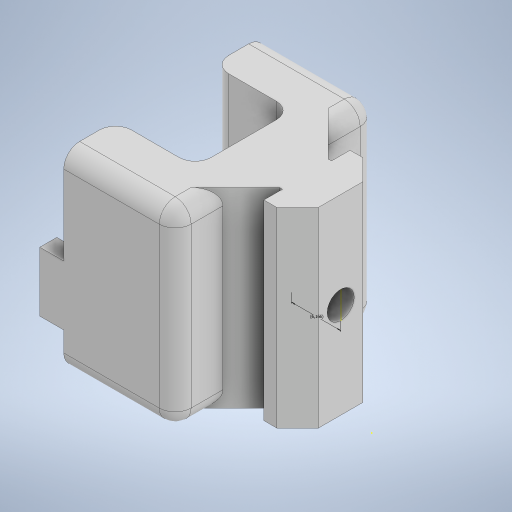
# Autodesk Inventor part: Montaż_kamery
Saved by Autodesk Inventor 2023 (Build 270158000, 158)
## iProperties
Created: 2023-04-17
Part Number: Montaż_kamery
Material: Ogólny
Document SubType Name: Modeling
Designer: janek
Density: 1 g/cm^3
Appearance: Domyślna
Author: janek
## iProperties of the stored document Montaż_kamery_Drukowanie 3D.ipt
Created: 2023-04-17
Part Number: Montaż_kamery_Drukowanie 3D
Material: Ogólny
Document SubType Name: Modeling
Designer: janek
Density: 1 g/cm^3
Appearance: Domyślna
Author: janek
Autodesk Inventor part; units mm, degrees
ref_plane "YZ Plane" through (0, 0, 0) normal (1, 0, 0) x (0, 1, 0)
ref_plane "XZ Plane" through (0, 0, 0) normal (0, 1, 0) x (-1, 0, 0)
ref_plane "XY Plane" through (0, 0, 0) normal (0, 0, 1) x (1, 0, 0)
sketch "Szkic3" plane through (0, 0, 0) normal (0, 1, 0) x (-1, 0, 0)
  line L0 (3.9, 2.7912) -> (3.9, -2.7912)
  line L1 (6.5152, 5.4063) -> (3.9, 2.7912)
  line L2 (8.1306, 5.4063) -> (6.5152, 5.4063)
  line L3 (8.1306, 5.4063) -> (8.1306, 3.0781)
  line L4 (8.1306, -3.0781) -> (8.1306, -5.4064)
  line L5 (8.1306, -5.4064) -> (6.5152, -5.4064)
  line L6 (6.5152, -5.4064) -> (3.9, -2.7912)
  line L7 (8.1306, 3.0781) -> (8.5306, 3.0781)
  line L8 (8.1306, -3.0781) -> (8.5306, -3.0781)
  line L9 (8.5306, -3.0781) -> (12.0661, -6.6136)
  line L10 (8.5306, 3.0781) -> (12.0661, 6.6136)
  line L11 (12.0661, -6.6136) -> (12.0661, -12.6136)
  line L12 (12.0661, 6.6136) -> (12.0661, 12.6136)
  line L13 (12.0661, 12.6136) -> (16.0661, 12.6136)
  line L14 (12.0661, -12.6136) -> (16.0661, -12.6136)
  line L15 (16.0661, -12.6136) -> (16.0661, 12.6136)
  point P0 (8.1306, 4.2422)
  dimension "d85" = 5.5823
  dimension "d88" = 135
  dimension "d89" = 135
  dimension "d90" = 1.6154
  dimension "d91" = 2.6152
  dimension "d92" = 2.3282
  dimension "d99" = 0.4
  dimension "d100" = 5
  dimension "d101" = 135
  dimension "d102" = 5
  dimension "d103" = 135
  dimension "d114" = 180
  dimension "d115" = 6
  dimension "d116" = 6
  dimension "d117" = 4
  dimension "d118" = 4
  constraints: 32 end point, 5 vertical, 4 equal length, 4 horizontal, 1 midpoint, 1 perpendicular, 1 other
  measures "d85" distance of L0.start L0.end
  measures "d88" angle of L6 L0
  measures "d89" angle of L1 L0
  measures "d90" distance of L4.end L5.end
  measures "d91" horizontal distance of L5.end L0.end
  measures "d92" distance of L4.start L4.end
  measures "d99" distance of L3.end L7.end
  measures "d100" distance of L8.end L9.end
  measures "d101" angle of L9 L8
  measures "d102" distance of L7.end L10.end
  measures "d103" angle of L7 L10
  measures "d114" angle of L2 L5
  measures "d115" distance of L9.end L11.end
  measures "d116" distance of L10.end L12.end
  measures "d117" distance of L12.end L13.end
  measures "d118" distance of L11.end L14.end
extrude "Wyciągnięcie proste1" add sketch "Szkic3" along normal blind 24
sketch "Szkic13" plane through (-16.0661, 0, -12.6136) normal (-1, 0, 0) x (0, 0, 1)
  line L0 (12.6136, 15.06) -> (15.2636, 13.53)
  line L1 (15.2636, 13.53) -> (15.2636, 10.47)
  line L2 (15.2636, 10.47) -> (12.6136, 8.94)
  line L3 (12.6136, 8.94) -> (9.9636, 10.47)
  line L4 (9.9636, 10.47) -> (9.9636, 13.53)
  line L5 (9.9636, 13.53) -> (12.6136, 15.06)
  line L6 (0, 24) -> (25.2273, 24) projected
  line L7 (25.2273, 0) -> (25.2273, 24) projected
  point P0 (12.6136, 0)
  point P1 (12.6136, 12)
  point P2 (12.6136, 24)
  dimension "d119" = 12
  dimension "d120" = 12.6136
  dimension "d121" = 5.3
  constraints: 12 end point, 1 midpoint, 1 parallel, 13 other
  measures "d119" distance of point (12.614, 24) point (12.614, 12)
  measures "d120" distance from line of L7 point (12.614, 12)
  measures "d121" distance between parallel lines of L1 L4
extrude "Wyciągnięcie proste5" cut sketch "Szkic13" against normal blind 6
sketch "Szkic14" plane through (-10.0661, 0, -12.6136) normal (-1, 0, 0) x (0, 0, 1)
  circle A0 centre (12.6136, 12) radius 1.7
  point P0 (12.6136, 0)
  dimension "d124" = 3.4
  constraints: 1 centre point
  measures "d124" diameter of A0
extrude "Wyciągnięcie proste6" cut sketch "Szkic14" against normal through all
sketch "Szkic15" plane through (0, 0, 0) normal (0, 0, 1) x (1, 0, 0)
  line L0 (-3.9, 13.7) -> (-3.9, 10.3) projected
  line L1 (-10.0661, 10.3) -> (-10.0661, 13.7) projected
  point P0 (0, 0)
  dimension "d127" = 6.1661
  measures "d127" distance between parallel lines of L1 L0
sketch "Szkic16" plane through (-16.0661, 0, -12.6136) normal (-1, 0, 0) x (0, 0, 1)
  point P0 (12.6136, 0)
sketch "Szkic17" plane through (-16.0661, 0, -12.6136) normal (-1, 0, 0) x (0, 0, 1)
  line L0 (25.2273, 0) -> (25.2273, 24) projected
  line L1 (0, 24) -> (25.2273, 24) projected
  line L2 (25.2273, 0) -> (18.7273, 0)
  line L3 (18.7273, 0) -> (18.7273, 24)
  line L4 (18.7273, 24) -> (25.2273, 24)
  line L5 (25.2273, 24) -> (25.2273, 0)
  line L6 (9.5355, 24) -> (6, 24) projected
  line L7 (6.5, 24) -> (0, 24)
  line L8 (0, 24) -> (0, 0)
  line L9 (0, 0) -> (6.5, 0)
  line L10 (6.5, 0) -> (6.5, 24)
  line L11 (0, 0) -> (0, 24) projected
  line L12 (0, 0) -> (25.2273, 0) projected
  point P0 (12.6136, 0)
  dimension "d128" = 6.5
  dimension "d129" = 6.5
  constraints: 16 end point, 5 parallel, 3 horizontal, 3 perpendicular, 2 point on line, 1 collinear
  measures "d128" distance of L3.end L4.end
  measures "d129" distance of L9.end L8.end
extrude "Wyciągnięcie proste7" add sketch "Szkic17" along normal blind 10 contours L2 L3 L1 L0 | L9 L8 L1 L10
sketch "Szkic18" plane through (-26.0661, 0, -12.6136) normal (-1, 0, 0) x (0, 0, 1)
  circle A0 centre (23.0973, 2) radius 0.85
  line L0 (25.2273, 0) -> (25.2273, 24) projected
  line L1 (18.7273, 0) -> (25.2273, 0) projected
  circle A1 centre (2.13, 2) radius 0.85
  line L2 (0, 0) -> (6.5, 0) projected
  line L3 (0, 24) -> (0, 0) projected
  circle A2 centre (23.0973, 14.5) radius 0.85
  circle A3 centre (2.13, 14.5) radius 0.85
  line L4 (2.13, 4.5) -> (0, 4.5)
  line L5 (0, 4.5) -> (0, 12)
  line L6 (0, 12) -> (2.13, 12)
  line L7 (2.13, 12) -> (2.13, 4.5)
  line L8 (25.2273, 0) -> (25.2273, 24) projected
  line L9 (25.2273, 4.5) -> (23.0973, 4.5)
  line L10 (23.0973, 4.5) -> (23.0973, 12)
  line L11 (23.0973, 12) -> (25.2273, 12)
  line L12 (25.2273, 12) -> (25.2273, 4.5)
  point P0 (12.6136, 0)
  point P1 (21.9773, 0)
  point P2 (0, 8.25)
  point P3 (2.13, 8.25)
  point P4 (0, 12)
  point P5 (0, 4.5)
  dimension "d132" = 1.7
  dimension "d133" = 2.13
  dimension "d134" = 2
  dimension "d135" = 2
  dimension "d136" = 2.13
  dimension "d137" = 1.7
  dimension "d138" = 1.7
  dimension "d139" = 12.5
  dimension "d140" = 2.13
  dimension "d141" = 1.7
  dimension "d142" = 2.13
  dimension "d143" = 12.5
  dimension "d144" = 2.5
  dimension "d145" = 2.5
  dimension "d147" = 2.13
  dimension "d148" = 2.5
  dimension "d149" = 2.5
  dimension "d150" = 2.13
  constraints: 16 end point, 4 centre point, 4 parallel, 3 midpoint, 2 horizontal, 2 perpendicular, 1 collinear, 1 point on line
  measures "d132" diameter of A0
  measures "d133" distance from line of L0 A0.centre
  measures "d134" vertical distance of point (21.977, 0) A0.centre
  measures "d135" distance from line of L2 A1.centre
  measures "d136" distance from line of A1.centre L3
  measures "d137" diameter of A1
  measures "d138" diameter of A2
  measures "d139" distance of A0.centre A2.centre
  measures "d140" distance from line of L0 A2.centre
  measures "d141" diameter of A3
  measures "d142" distance from line of L3 A3.centre
  measures "d143" distance of A1.centre A3.centre
  measures "d144" distance of L6.end A3.centre
  measures "d145" distance of A1.centre L4.start
  measures "d147" distance between parallel lines of L5 L7
  measures "d148" distance of A0.centre L9.end
  measures "d149" distance of A2.centre L10.end
  measures "d150" distance between parallel lines of L10 L0
extrude "Wyciągnięcie proste8" add sketch "Szkic18" along normal blind 3 contours L9 L10 L11 L0 | L6 L7 L4 L3
extrude "Wyciągnięcie proste9" cut sketch "Szkic18" against normal blind 5 contours A0 | A1 | A2 | A3
fillet "Zaokrąglenie1" radius 2 14 edges at (-16.0661, 12, 6.1136) (-16.0661, 12, -6.1136) (-26.0661, 12, -6.1136) (-26.0661, 12, 6.1136) (-12.0661, 12, 12.6136) (-12.0661, 12, -12.6136) (-19.0661, 0, -12.6136) (-12.0661, 0, -9.6136) (-19.0661, 24, -12.6136) (-12.0661, 24, -9.6136) (-12.0661, 24, 9.6136) (-19.0661, 24, 12.6136) (-12.0661, 0, 9.6136) (-19.0661, 0, 12.6136)
